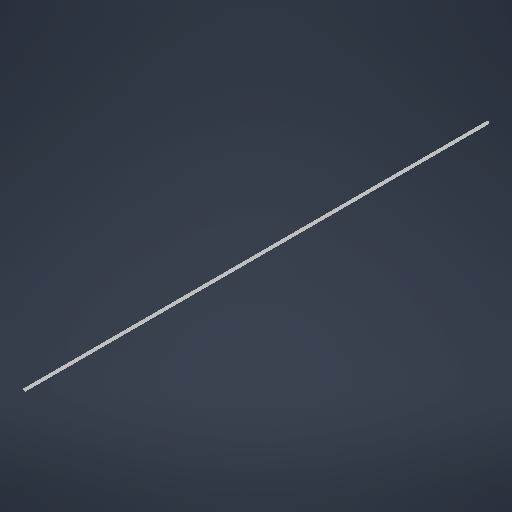
# Autodesk Inventor part: SP40-02 JUNTA INT CRISTAL 1987ç mm
Saved by Autodesk Inventor 2025 (Build 290162000, 162)
## iProperties
Created: 2026-01-18
Part Number: SP40-02 JUNTA INT CRISTAL 1987ç mm
Material: Caucho
Document SubType Name: Modeling
Designer: ROLANDO
Density: 0.93 g/cm^3
Appearance: Caucho - Negro
Author: ROLANDO
Autodesk Inventor part; units mm, degrees
ref_plane "YZ Plane" through (0, 0, 0) normal (1, 0, 0) x (0, 1, 0)
ref_plane "XZ Plane" through (0, 0, 0) normal (0, 1, 0) x (-1, 0, 0)
ref_plane "XY Plane" through (0, 0, 0) normal (0, 0, 1) x (1, 0, 0)
sketch "Boceto3" plane through (0, 0, 0) normal (0, 0, 1) x (1, 0, 0)
  line L0 (-13.5546, 31.7799) -> (-18.7766, 31.7799)
  line L1 (-12.1166, 33.1799) -> (-12.1166, 30.6799)
  line L2 (-12.1166, 30.6799) -> (-12.8266, 30.6799)
  line L3 (-12.8266, 30.6799) -> (-13.5546, 31.7799)
  arc A0 (-18.7766, 31.7799) -> (-21.5166, 29.0399) centre (-18.7766, 29.0399) ccw
  line L4 (-12.1166, 33.1799) -> (-8.6166, 33.1799)
  line L5 (-21.5166, 29.0399) -> (-21.5166, 26.2799)
  arc A1 (-8.6166, 33.1799) -> (-8.6166, 26.2799) centre (6.7872, 29.7299) ccw
  line L6 (-21.5166, 26.2799) -> (-21.0166, 26.2799)
  line L7 (-8.6166, 26.2799) -> (-9.1166, 26.2799)
  line L8 (-8.6166, 38.7215) -> (-8.6166, 22.0906) construction
  arc A2 (-9.1166, 26.2799) -> (-21.0166, 26.2799) centre (-15.0666, 20.0463) ccw
  dimension "d218" = 2.5
  dimension "d219" = 0.71
  dimension "d221" = 33.5
  dimension "d223" = 2.74
  dimension "d281" = 3.5
  dimension "d288" = 2.76
  dimension "d291" = 0.5
  dimension "d292" = 0.5
  dimension "d301" = 5.2219
  constraints: 18 end point, 6 point on circle, 3 centre point, 3 horizontal, 3 vertical, 2 point on line, 1 collinear, 1 perpendicular, 1 tangent
  measures "d218" distance of L1.start L1.end
  measures "d219" distance of L1.end L2.end
  measures "d221" angle of L1 L3
  measures "d223" radius of A0
  measures "d281" distance of L1.start L4.end
  measures "d288" distance of L5.start L5.end
  measures "d291" distance of L5.end L6.end
  measures "d292" distance of L7.start L7.end
  measures "d301" distance of L0.start L0.end
extrude "Extrusión4" add sketch "Boceto3" against normal blind 3000
ref_plane "Plano de trabajo2" through (-8.6166, 33.1799, 0) normal (-1, 0, 0) x (0, 0, -1)
ref_plane "Plano de trabajo4" through (0, 0, -1500) normal (0, 0, 1) x (1, 0, 0)
sketch "Boceto5" plane through (-8.6166, 33.1799, 0) normal (-1, 0, 0) x (0, 0, -1)
  line L0 (0, 0) -> (0, 6.9) projected
  line L1 (0, 0) -> (3000, 0) projected
  line L2 (6.9, 0) -> (0, 0)
  line L3 (0, 0) -> (0, 6.9)
  line L4 (0, 6.9) -> (3000, 6.9) projected
  line L5 (0, 6.9) -> (6.9, 0)
  point P0 (0, 0)
  dimension "d300" = 45
  constraints: 6 end point, 1 horizontal, 1 perpendicular, 1 point on line
  measures "d300" angle of L0 L5
extrude "Extrusión6" cut sketch "Boceto5" along normal through all
